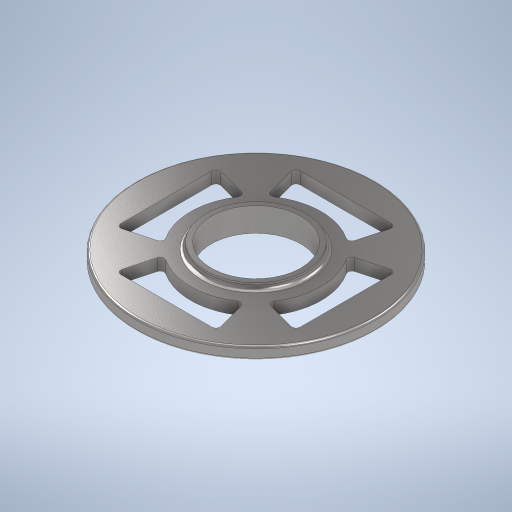
# Autodesk Inventor part: practice6
Saved by Autodesk Inventor 2024 (Build 280153000, 153)
## iProperties
Created: 2024-02-15
Part Number: practice6
Material: Stahl, galvanisiert
Document SubType Name: Modeling
Designer: ffogue
Density: 7.85 g/cm^3
Appearance: Galvanisiert
Author: ffogue
Autodesk Inventor part; units mm, degrees
ref_plane "YZ Plane" through (0, 0, 0) normal (1, 0, 0) x (0, 1, 0)
ref_plane "XZ Plane" through (0, 0, 0) normal (0, 1, 0) x (-1, 0, 0)
sketch "Skizze1" plane through (0, 0, 0) normal (0, 0, 1) x (1, 0, 0)
  circle A0 centre (0, 0) radius 60
  dimension "d0" = 120
  constraints: 1 centre point, 1 coincident
  measures "d0" diameter of A0
extrude "Extrusion1" add sketch "Skizze1" along normal blind 6
ref_plane "Arbeitsebene1" through (0, 0, 3) normal (0, 0, 1) x (1, 0, 0)
sketch "Skizze3" plane through (0, 0, 3) normal (0, 0, 1) x (1, 0, 0)
  circle A0 centre (0, 0) radius 25
  dimension "d5" = 50
  constraints: 1 centre point, 1 coincident
  measures "d5" diameter of A0
extrude "Extrusion2" add sketch "Skizze3" along normal mid plane 12
sketch "Skizze4" plane through (0, 0, 9) normal (0, 0, 1) x (1, 0, 0)
  circle A0 centre (0, 0) radius 22.5
  dimension "d8" = 45
  constraints: 1 centre point, 1 coincident
  measures "d8" diameter of A0
extrude "Extrusion3" cut sketch "Skizze4" against normal blind 12
fillet "Rundung1" radius 2 1 edges at (-25, 0, 6)
fillet "Rundung2" radius 2 1 edges at (-25, 0, 0)
sketch "Skizze5" plane through (0, 0, 6) normal (0, 0, 1) x (1, 0, 0)
  line L0 (25.4807, -45) -> (-25.4807, -45)
  arc A0 (-20.3044, -25.6815) -> (20.3044, -25.6815) centre (0, 0) ccw
  circle A1 centre (0, 0) radius 27 projected
  line L1 (20.3044, -25.6815) -> (25.4807, -45)
  line L2 (-20.3044, -25.6815) -> (-25.4807, -45)
  line L3 (0, 0) -> (0, -59.7048) construction
  circle A2 centre (0, 0) radius 22.5 projected
  dimension "d16" = 20
  dimension "d17" = 45
  dimension "d18" = 75
  constraints: 8 end point, 2 concentric, 2 point on circle, 1 centre point, 1 horizontal, 1 symmetric about line, 1 vertical
  measures "d16" distance of L1.start L0.start
  measures "d17" distance from line of point (0, 0) L0
  measures "d18" angle of L0 L1
extrude "Extrusion4" cut sketch "Skizze5" against normal blind 12 contours L0 L2 A0 L1
fillet "Rundung3" radius 2 2 edges at (-25.4807, -45, 3) (25.4807, -45, 3)
fillet "Rundung4" radius 2 2 edges at (-20.3044, -25.6815, 3) (20.3044, -25.6815, 3)
pattern_circular "Runde Anordnung1" count 4 over 360 about axis through (0, 0, 0) along (0, 0, 1) of "Extrusion4", "Rundung4", "Rundung3"
fillet "Rundung5" radius 1 2 edges at (-60, 0, 0) (-60, 0, 6)
